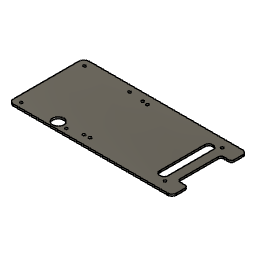
board mount v10 (Autodesk Fusion 360 design; units mm, degrees)
Autodesk Fusion 360 part; units mm, degrees
sketch "Sketch1" plane through (0, 0, 0) normal (0, 0, 1) x (1, 0, 0)
  line L0 (-46.9876, 42.1313) -> (126.9807, 42.1313)
  line L1 (126.9807, -42.8687) -> (-48.0193, -42.8687)
  line L2 (-53.0193, -37.8687) -> (-53.0193, 36.0996)
  arc A0 (-46.9876, 42.1313) -> (-53.0193, 36.0996) centre (-46.9876, 36.0996) ccw
  circle A1 centre (22.0901, -32.8649) radius 1.5
  circle A2 centre (22.6428, 33.2081) radius 1.5
  line L3 (51.8879, 20.2448) -> (51.8879, 20.5459)
  arc A3 (131.9807, 37.1313) -> (126.9807, 42.1313) centre (126.9807, 37.1313) ccw
  arc A4 (126.9807, -42.8687) -> (131.9807, -37.8687) centre (126.9807, -37.8687) ccw
  circle A5 centre (-45.079, 34.8744) radius 1.5
  circle A6 centre (5.921, 34.8744) radius 1.5
  circle A7 centre (-45.079, -36.8256) radius 1.5
  circle A8 centre (5.921, -36.8256) radius 1.5
  arc A9 (-53.0193, -37.8687) -> (-48.0193, -42.8687) centre (-48.0193, -37.8687) ccw
  line L4 (104.9268, 30.2898) -> (105.5, 30.2898)
  line L5 (110, 25.7898) -> (110, -25.5)
  line L6 (105.5, -30) -> (104.9268, -30)
  line L7 (100.4268, -25.5) -> (100.4268, 25.7898)
  arc A10 (104.9268, 30.2898) -> (100.4268, 25.7898) centre (104.9268, 25.7898) ccw
  arc A11 (110, 25.7898) -> (105.5, 30.2898) centre (105.5, 25.7898) ccw
  arc A12 (100.4268, -25.5) -> (104.9268, -30) centre (104.9268, -25.5) ccw
  arc A13 (105.5, -30) -> (110, -25.5) centre (105.5, -25.5) ccw
  line L8 (128.9807, 24.5178) -> (123, 24.5178)
  line L9 (120, 21.5178) -> (120, -22)
  line L10 (123, -25) -> (128.9807, -25)
  line L11 (131.9807, 37.1313) -> (131.9807, 27.5178)
  line L12 (131.9807, -28) -> (131.9807, -37.8687)
  arc A14 (128.9807, 24.5178) -> (131.9807, 27.5178) centre (128.9807, 27.5178) ccw
  arc A15 (123, 24.5178) -> (120, 21.5178) centre (123, 21.5178) ccw
  arc A16 (120, -22) -> (123, -25) centre (123, -22) ccw
  arc A17 (131.9807, -28) -> (128.9807, -25) centre (128.9807, -28) ccw
  circle A18 centre (-5.5632, -34.5538) radius 6.5
  circle A19 centre (113.4506, 32.5907) radius 1.5
  circle A20 centre (113.4506, -32.3271) radius 1.5
  circle A21 centre (28.5327, -32.3271) radius 1.5
  circle A22 centre (28.5327, 32.5907) radius 1.5
  point P0 (-53.0193, 42.1313)
  point P1 (114.0401, 42.1313)
  point P2 (-53.0193, -42.8687)
  point P3 (-68.019, -42.783)
  point P4 (-66.7458, 12.2022)
  point P5 (131.9807, -42.8687)
  dimension "d6" = 85
  dimension "d7" = 15
  dimension "d8" = 55
  dimension "d67" = 3
  dimension "d69" = 3
  dimension "d120" = 5
  dimension "d147" = 51
  dimension "d148" = 71.7
  dimension "d149" = 3
  dimension "d150" = 3
  dimension "d151" = 3
  dimension "d152" = 3
  dimension "d170" = 5
  dimension "d177" = 4.5
  dimension "d183" = 3
  dimension "d184" = 13
  dimension "d190" = 3
  dimension "d191" = 3
  dimension "d192" = 3
  dimension "d193" = 3
  constraint horizontal L0
  constraint horizontal L1
  constraint vertical L2
  constraint coincident P1 L0
  constraint coincident P0 L0
  constraint coincident P0 L2
  constraint tangent L0 A0
  constraint tangent L2 A0
  constraint coincident P2 L2
  constraint tangent L0 A3
  constraint coincident L1 P5
  constraint tangent L1 A4
  constraint equal A3 A4
  constraint coincident P2 L1
  constraint tangent L2 A9
  constraint tangent L1 A9
  constraint horizontal L4
  constraint vertical L5
  constraint horizontal L6
  constraint vertical L7
  constraint tangent L4 A10
  constraint tangent L7 A10
  constraint tangent L4 A11
  constraint tangent L5 A11
  constraint equal A10 A11
  constraint tangent L7 A12
  constraint tangent L6 A12
  constraint equal A10 A12
  constraint tangent L5 A13
  constraint tangent L6 A13
  constraint equal A10 A13
  constraint horizontal L8
  constraint vertical L9
  constraint horizontal L10
  constraint tangent A3 L11
  constraint perpendicular L8 L11
  constraint tangent A4 L12
  constraint tangent L11 A14
  constraint tangent L8 A14
  constraint tangent L8 A15
  constraint tangent L9 A15
  constraint equal A14 A15
  constraint tangent L9 A16
  constraint tangent L10 A16
  constraint equal A14 A16
  constraint tangent L10 A17
  constraint tangent L12 A17
  constraint equal A14 A17
  measures "d6" distance of P0 P2
  measures "d7" distance of P2 P3
  measures "d8" distance of P3 P4
  measures "d67" diameter of A1
  measures "d69" diameter of A2
  measures "d120" radius of A3
  measures "d147" distance of A5.centre A6.centre
  measures "d148" distance of A5.centre A7.centre
  measures "d149" diameter of A5
  measures "d150" diameter of A6
  measures "d151" diameter of A7
  measures "d152" diameter of A8
  measures "d170" radius of A9
  measures "d177" radius of A10
  measures "d183" radius of A14
  measures "d184" diameter of A18
  measures "d190" diameter of A19
  measures "d191" diameter of A20
  measures "d192" diameter of A21
  measures "d193" diameter of A22
extrude "Extrude18" add sketch "Sketch1" along normal blind 2
